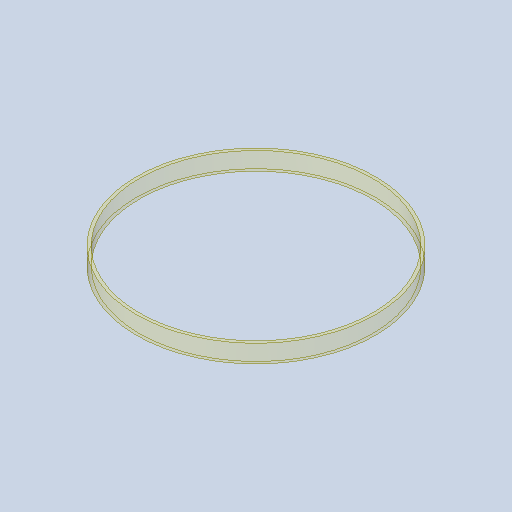
# Autodesk Inventor part: TorsOsc-202511-cell-wall
Saved by Autodesk Inventor 2026 (Build 300175050, 175E)
## iProperties
Created: 2025-12-02
Part Number: TorsOsc-202511-cell-wall
Material: Epoxy Resin
Document SubType Name: Modeling
Designer: schanen
Density: 1.14 g/cm^3
Appearance: Clear - Yellow
Mass: 2.11879 g
Surface Area: 34.7906 cm^2
Volume: 1.61739 cm^3
Author: schanen
Autodesk Inventor part; units mm, degrees
ref_plane "YZ Plane" through (0, 0, 0) normal (1, 0, 0) x (0, 1, 0)
ref_plane "XZ Plane" through (0, 0, 0) normal (0, 1, 0) x (-1, 0, 0)
ref_plane "XY Plane" through (0, 0, 0) normal (0, 0, 1) x (1, 0, 0)
sketch "Sketch1" plane through (0, 0, 0) normal (1, 0, 0) x (0, 1, 0)
  line L0 (0, 20) -> (3, 20)
  line L1 (3, 20) -> (3, 19.5)
  line L2 (3, 19.5) -> (0, 19.5)
  line L3 (0, 20) -> (0, 19.5)
  line L4 (-1.8, 0) -> (3.8, 0) projected
  point P0 (0, 0)
  point P1 (-1, 3.5)
  dimension "d0" = 3
  dimension "d3" = 0.5
  dimension "d17" = 20
  constraints: 8 end point, 2 perpendicular, 1 vertical, 1 vertical alignment
  measures "d0" distance of L0.start L0.end
  measures "d3" distance of L0.end L1.end
  measures "d17" distance between parallel lines of L4 L0
revolve "Revolution2" add sketch "Sketch1" angle 360 about axis through (0, -10, 0) along (0, 1, 0)
body "Solid2"
